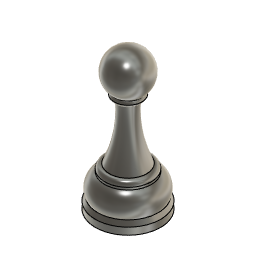
Sketch26_Final v1 (Autodesk Fusion 360 design; units mm, degrees)
Autodesk Fusion 360 part; units mm, degrees
sketch "Sketch1" plane through (0, 0, 0) normal (0, 1, 0) x (1, 0, 0)
  line L0 (0, 0) -> (0, -60)
  line L1 (0, -60) -> (0, -51)
  circle A0 centre (0, -51) radius 9
  line L2 (50, -60) -> (50, 0)
  line L3 (25, -60) -> (25, -44.29)
  line L4 (5.998, -44.29) -> (-4.0005, -44.29)
  line L5 (5.998, -44.29) -> (5.998, -41.03)
  line L6 (5.998, -41.03) -> (-3.9995, -41.03)
  arc A1 (-3.9995, -41.03) -> (-5.9655, -42.6624) centre (-3.9995, -43.03) ccw
  arc A2 (-5.9655, -42.6624) -> (-4.0005, -44.29) centre (-4.0005, -42.29) ccw
  line L7 (0, -41.03) -> (0, -16.97)
  line L8 (0, 0) -> (14, 0)
  line L9 (14, 0) -> (-14, 0)
  line L10 (-14, 0) -> (-14, -3)
  line L11 (-14, -3) -> (14, -3)
  line L12 (14, -3) -> (14, 0)
  line L13 (0, -3) -> (0, -5)
  line L14 (0, -5) -> (13, -5)
  line L15 (13, -5) -> (-13, -5)
  line L16 (13, -5) -> (14, -3)
  line L17 (-13, -5) -> (-14, -3)
  line L18 (0, -5) -> (0, -13.97)
  line L19 (0, -13.97) -> (10, -13.97)
  line L20 (10, -13.97) -> (-10, -13.97)
  line L21 (-10, -13.97) -> (-10, -14.97)
  line L22 (-10, -14.97) -> (10, -14.97)
  line L23 (10, -14.97) -> (10, -13.97)
  arc A3 (-13, -5) -> (-10, -13.97) centre (-6.6188, -7.8525) ccw
  line L24 (8, -16.97) -> (-8, -16.97)
  arc A4 (-10, -14.97) -> (-8, -16.97) centre (-8, -14.97) ccw
  arc A5 (-3.9995, -41.03) -> (-8, -16.97) centre (-53.8331, -36.9532) ccw
  line L25 (0, 0) -> (0, -65)
  point P0 (-6.002, -41.03)
  dimension "d1" = 60
  dimension "d3" = 9
  dimension "d4" = 18
  dimension "d5" = 15.71
  dimension "d6" = 3.26
  dimension "d7" = 12
  dimension "d8" = 2
  dimension "d9" = 2
  dimension "d10" = 24.06
  dimension "d12" = 14
  dimension "d14" = 3
  dimension "d15" = 28
  dimension "d16" = 2
  dimension "d17" = 13
  dimension "d18" = 26
  dimension "d19" = 8.97
  dimension "d20" = 10
  dimension "d21" = 20
  dimension "d22" = 1
  dimension "d23" = 8
  dimension "d24" = 16
  dimension "d25" = 2
  dimension "d26" = 50
  constraint coincident L0.start L8.start
  constraint vertical L0
  constraint parallel L0 L1
  constraint coincident L1.end A0.centre
  constraint vertical L2
  constraint vertical L3
  constraint perpendicular L0 L4
  constraint coincident A0 L4.start
  constraint perpendicular L4 L5
  constraint perpendicular L0 L6
  constraint coincident P0 L6
  constraint tangent L6 A1
  constraint tangent L4 A2
  constraint coincident L0 L7.start
  constraint coincident L6 L7.start
  constraint perpendicular L6 L7
  constraint perpendicular L0 L8
  constraint parallel L8 L9
  constraint perpendicular L9 L10
  constraint perpendicular L0 L11
  constraint midpoint L11 L13.start
  constraint perpendicular L11 L13
  constraint perpendicular L0 L14
  constraint perpendicular L13 L15
  constraint perpendicular L14 L18
  constraint perpendicular L0 L19
  constraint parallel L19 L20
  constraint perpendicular L20 L21
  constraint perpendicular L21 L22
  constraint perpendicular L7 L24
  constraint tangent L21 A4
  constraint tangent L24 A4
  constraint perpendicular L8 L25
  measures "d1" distance of L0.start L0.end
  measures "d3" distance of L0.end L1.end
  measures "d4" diameter of A0
  measures "d5" distance of L3.start L3.end
  measures "d6" distance of L4.start L5.end
  measures "d7" distance of L5.end P0
  measures "d8" radius of A1
  measures "d9" radius of A2
  measures "d10" distance of L7.start L7.end
  measures "d12" distance of L0.start L8.end
  measures "d14" distance of L9.end L10.end
  measures "d15" distance of L10.end L11.end
  measures "d16" distance of L13.start L13.end
  measures "d17" distance of L13.end L14.end
  measures "d18" distance of L14.end L15.end
  measures "d19" distance of L13.end L18.end
  measures "d20" distance of L18.end L19.end
  measures "d21" distance of L19.end L20.end
  measures "d22" distance of L20.end L21.end
  measures "d23" distance of L7.end L24.start
  measures "d24" distance of L24.start L24.end
  measures "d25" radius of A4
  measures "d26" radius of A5
revolve "Revolve1" add sketch "Sketch1" angle 360 about axis through (0, 0, 0) along (0, 0, 1) second angle 360 contours L0 L9 L10 L11 L25 | L0 L11 L13 L15 L17 L25 | L0 L15 L18 L20 A3 L25 | L0 L20 L21 L22 L25 | L0 L22 L24 A4 L25 | L0 L6 L7 L24 A5 L25 | L0 A0 L6 A1 A2 L25 | L0 L1 A0 L4 A2 L25
